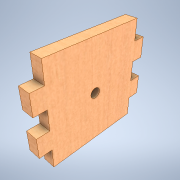
# Autodesk Inventor part: FRONT V2
Saved by Autodesk Inventor 2021.2 (Build 252289000, 289)
## iProperties
Created: 2021-03-11
Part Number: FRONT V2
Material: Wood (Cherry)
Document SubType Name: Modeling
Designer: 443201246
Density: 0.63 g/cm^3
Appearance: Cherry - Natural Low Gloss
Author: 443201246
Autodesk Inventor part; units mm, degrees
ref_plane "YZ Plane" through (0, 0, 0) normal (1, 0, 0) x (0, 1, 0)
ref_plane "XZ Plane" through (0, 0, 0) normal (0, 1, 0) x (-1, 0, 0)
ref_plane "XY Plane" through (0, 0, 0) normal (0, 0, 1) x (1, 0, 0)
sketch "Sketch6" plane through (0, 0, 0) normal (1, 0, 0) x (0, 1, 0)
  line L0 (-50, 59.5) -> (50, 59.5)
  line L1 (50, 59.5) -> (50, -59.5)
  line L2 (50, -59.5) -> (-50, -59.5)
  line L3 (-50, -59.5) -> (-50, 59.5)
  line L4 (-50, 59.5) -> (50, -59.5) construction
  line L5 (50, 59.5) -> (-50, -59.5) construction
  point P0 (0, 0)
  dimension "d28" = 100
  dimension "d29" = 119
  constraints: 12 end point, 2 midpoint, 2 parallel, 1 horizontal, 1 perpendicular
  measures "d28" distance of L1.end L2.end
  measures "d29" distance of L0.end L1.end
extrude "Extrusion5" add sketch "Sketch6" along normal mid plane 12
sketch "Sketch7" plane through (6, 0, 0) normal (1, 0, 0) x (0, 0, -1)
  line L0 (-59.5, 50) -> (-59.5, -50) projected
  line L1 (-59.5, -50) -> (-47.5, -50)
  line L2 (-47.5, -50) -> (-47.5, -30)
  line L3 (-47.5, -30) -> (-59.5, -30)
  line L4 (-59.5, -30) -> (-59.5, -50)
  line L5 (-59.5, -50) -> (-59.5, 50) projected
  line L6 (-59.5, -10) -> (-47.5, -10)
  line L7 (-47.5, -10) -> (-47.5, 10)
  line L8 (-47.5, 10) -> (-59.5, 10)
  line L9 (-59.5, 10) -> (-59.5, -10)
  line L10 (-59.5, 30) -> (-47.5, 30)
  line L11 (-47.5, 30) -> (-47.5, 50)
  line L12 (-47.5, 50) -> (-59.5, 50)
  line L13 (-59.5, 50) -> (-59.5, 30)
  point P0 (0, 0)
  dimension "d32" = 12
  dimension "d33" = 20
  dimension "d34" = 12
  dimension "d35" = 20
  dimension "d36" = 20
  dimension "d39" = 12
  dimension "d40" = 20
  dimension "d41" = 20
  constraints: 24 end point, 6 parallel, 3 horizontal, 3 perpendicular, 2 point on line
  measures "d32" distance of L3.end L2.end
  measures "d33" distance of L2.end L1.end
  measures "d34" distance of L8.end L7.end
  measures "d35" distance of L7.end L6.end
  measures "d36" distance between parallel lines of L6 L3
  measures "d39" distance of L12.end L11.end
  measures "d40" distance of L11.end L10.end
  measures "d41" distance between parallel lines of L10 L8
extrude "Extrusion6" cut sketch "Sketch7" against normal through all
mirror "Mirror2" about plane through (0, 0, 0) normal (0, 0, 1) of "Extrusion6"
sketch "Sketch8" plane through (6, 0, 0) normal (1, 0, 0) x (0, 0, -1)
  circle A0 centre (0, 0) radius 5
  dimension "d44" = 10
  constraints: 1 centre point, 1 coincident
  measures "d44" diameter of A0
extrude "Extrusion7" cut sketch "Sketch8" against normal through all
body "Solid2"
